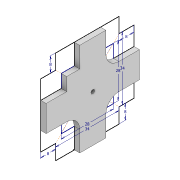
# Autodesk Inventor part: Cube_Insert_Motion_adapter_srew_back
Saved by Autodesk Inventor 2022 (Build 260153000, 153)
## iProperties
Created: 2023-06-30
Part Number: Cube_Insert_Motion_adapter_srew_back
Material: Generisch
Document SubType Name: Modeling
Designer: UC2
Density: 1 g/cm^3
Appearance: Vorgabe
Author: UC2
Autodesk Inventor part; units mm, degrees
ref_plane "YZ Plane" through (0, 0, 0) normal (1, 0, 0) x (0, 1, 0)
ref_plane "XZ Plane" through (0, 0, 0) normal (0, 1, 0) x (-1, 0, 0)
ref_plane "XY Plane" through (0, 0, 0) normal (0, 0, 1) x (1, 0, 0)
sketch "Skizze1" plane through (0, 0, 0) normal (1, 0, 0) x (0, 1, 0)
  line L0 (14, 14) -> (-14, 14)
  line L1 (-14, 14) -> (-14, -14)
  line L2 (-14, -14) -> (14, -14)
  line L3 (14, -14) -> (14, 14)
  line L4 (14, 14) -> (-14, -14) construction
  line L5 (-14, 14) -> (14, -14) construction
  line L6 (17, 17) -> (-17, -17) construction
  line L7 (-17, 17) -> (17, -17) construction
  line L8 (-17, 17) -> (-17, 25)
  line L9 (-17, 25) -> (17, 25)
  line L10 (17, 25) -> (17, 17)
  line L11 (17, 17) -> (25, 17)
  line L12 (25, 17) -> (25, -17)
  line L13 (25, -17) -> (17, -17)
  line L14 (17, -17) -> (17, -25)
  line L15 (17, -25) -> (-17, -25)
  line L16 (-17, -25) -> (-17, -17)
  line L17 (-17, -17) -> (-25, -17)
  line L18 (-25, -17) -> (-25, 17)
  line L19 (-25, 17) -> (-17, 17)
  line L20 (-7, 14) -> (-7, 25)
  line L21 (7, 14) -> (7, 25)
  line L22 (14, 7) -> (25, 7)
  line L23 (14, -7) -> (25, -7)
  line L24 (7, -14) -> (7, -25)
  line L25 (-7, -14) -> (-7, -25)
  line L26 (-14, -7) -> (-25, -7)
  line L27 (-14, 7) -> (-25, 7)
  point P0 (0, 0)
  dimension "d0" = 28
  dimension "d1" = 28
  dimension "d2" = 34
  dimension "d3" = 34
  dimension "d4" = 8
  dimension "d5" = 8
  dimension "d6" = 8
  dimension "d7" = 8
  constraints: 56 end point, 18 point on line, 14 perpendicular, 4 midpoint, 3 horizontal, 3 vertical, 2 parallel
  measures "d0" distance of L2.end L1.end
  measures "d1" distance of L1.end L0.end
  measures "d2" distance of L7.end L6.end
  measures "d3" distance of L6.end L7.start
  measures "d4" distance of L7.start L8.end
  measures "d5" distance of L6.start L11.end
  measures "d6" distance of L7.end L14.end
  measures "d7" distance of L17.start L17.end
extrude "Extrusion1" add sketch "Skizze1" along normal blind 3 contours L3 L2 L1 L0 | L0 L20 L9 L21 | L22 L12 L23 L3 | L1 L26 L18 L27 | L24 L15 L25 L2
hole "Bohrung1" at (0, 14, -14) at (0, -14, -14) at (0, -14, 14) direction (1, 0, 0) diameter 14 end through all
hole "Bohrung2" at (0, 0, 0) direction (1, 0, 0) diameter 2 end through all
